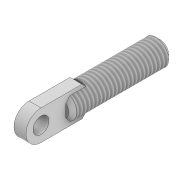
# Autodesk Inventor part: Break_Tensor
Saved by Autodesk Inventor 2020 (Build 240168000, 168)
## iProperties
Created: 2020-02-19
Part Number: Break_Tensor
Material: Generic
Document SubType Name: Modeling
Designer: Charlie
Density: 1 g/cm^3
Appearance: Default
Author: Charlie
Autodesk Inventor part; units mm, degrees
ref_plane "YZ Plane" through (0, 0, 0) normal (1, 0, 0) x (0, 1, 0)
ref_plane "XZ Plane" through (0, 0, 0) normal (0, 1, 0) x (-1, 0, 0)
ref_plane "XY Plane" through (0, 0, 0) normal (0, 0, 1) x (1, 0, 0)
sketch "Sketch1" plane through (0, 0, 0) normal (0, 0, 1) x (1, 0, 0)
  circle A0 centre (0, 0) radius 6.35
  dimension "d0" = 12.7
  constraints: 1 centre point, 1 coincident
  measures "d0" diameter of A0
extrude "Extrusion1" add sketch "Sketch1" along normal mid plane 50
sketch "Sketch2" plane through (0, 0, 25) normal (0, 0, 1) x (1, 0, 0)
  line L0 (-3, -13.1035) -> (3, -13.1035)
  line L1 (3, -13.1035) -> (3, 13.1035)
  line L2 (3, 13.1035) -> (-3, 13.1035)
  line L3 (-3, 13.1035) -> (-3, -13.1035)
  line L4 (-3, -13.1035) -> (3, 13.1035) construction
  line L5 (3, -13.1035) -> (-3, 13.1035) construction
  point P0 (0, 0)
  dimension "d3" = 6
  constraints: 12 end point, 2 midpoint, 2 parallel, 1 horizontal, 1 perpendicular
  measures "d3" distance of L2.end L1.end
extrude "Extrusion2" cut sketch "Sketch2" against normal blind 10
sketch "Sketch3" plane through (0, 0, 15) normal (0, 0, 1) x (1, 0, 0)
  line L0 (-3, -7.5) -> (3, -7.5)
  line L1 (3, -7.5) -> (3, 7.5)
  line L2 (3, 7.5) -> (-3, 7.5)
  line L3 (-3, 7.5) -> (-3, -7.5)
  line L4 (-3, -7.5) -> (3, 7.5) construction
  line L5 (3, -7.5) -> (-3, 7.5) construction
  point P0 (0, 0)
  dimension "d6" = 6
  dimension "d7" = 15
  constraints: 12 end point, 2 midpoint, 2 parallel, 1 horizontal, 1 perpendicular
  measures "d6" distance of L2.end L1.end
  measures "d7" distance of L1.end L0.end
extrude "Extrusion3" add sketch "Sketch3" along normal blind 30 separate body
fillet "Fillet1" radius 7.5 2 edges at (0, 7.5, 45) (0, -7.5, 45)
thread "Thread1" size "1/2-13 UNC" class "2A" standard "ANSI Unified Screw Threads" full length
chamfer "Chamfer1" distance 2 angle 45 1 edges at (-6.35, 0, -25)
sketch "Sketch5" plane through (-3, -7.5, 15) normal (-1, 0, 0) x (0, 0, 1)
  arc A0 (22.5, 0) -> (22.5, 15) centre (22.5, 7.5) ccw projected
  line L0 (0, 15) -> (22.5, 15) projected
  line L1 (0, 15) -> (0, 0) projected
  line L2 (0, 0) -> (22.5, 0) projected
  circle A1 centre (22.5, 7.5) radius 4
  point P0 (-15, 7.5)
  dimension "d20" = 8
  constraints: 1 centre point, 1 coincident
  measures "d20" diameter of A1
extrude "Extrusion5" cut sketch "Sketch5" against normal through all contours A1 bodies 2
chamfer "Chamfer2" distance 2 angle 45 3 edges at (-6.35, 0, 25) (5.4485, -3.2613, 25) (5.4485, 3.2613, 25)
chamfer "Chamfer3" distance 2 angle 45 2 edges at (0, -7.5, 15) (0, 7.5, 15)
body "Solid1"
body "Solid2"
